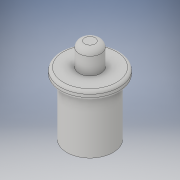
# Autodesk Inventor part: ConexionDireccionTop
Saved by Autodesk Inventor 2019 (Build 230136000, 136)
## iProperties
Created: 2019-12-22
Part Number: ConexionDireccionTop
Material: Generic
Document SubType Name: Modeling
Designer: Sergio
Density: 1 g/cm^3
Appearance: Default
Author: Sergio
Autodesk Inventor part; units mm, degrees
ref_plane "YZ Plane" through (0, 0, 0) normal (1, 0, 0) x (0, 1, 0)
ref_plane "XZ Plane" through (0, 0, 0) normal (0, 1, 0) x (-1, 0, 0)
ref_plane "XY Plane" through (0, 0, 0) normal (0, 0, 1) x (1, 0, 0)
sketch "Sketch1" plane through (0, 0, 0) normal (1, 0, 0) x (0, 1, 0)
  line L0 (30.0226, 0) -> (0.0226, 0)
  line L1 (0.0226, -8.15) -> (19.0226, -8.15)
  line L2 (19.0226, -8.15) -> (19.0226, -10.35)
  line L3 (19.0226, -10.35) -> (22.0226, -10.35)
  line L4 (22.0226, -10.35) -> (22.0226, -3.85)
  line L5 (22.0226, -3.85) -> (30.0226, -3.85)
  line L6 (30.0226, -3.85) -> (30.0226, 0)
  line L7 (0.0226, 0) -> (0.0226, -8.15)
  line L8 (50.327, 0) -> (-8.0634, 0) construction
  point P0 (0, 0)
  dimension "d0" = 3.85
  dimension "d2" = 3
  dimension "d3" = 6.5
  dimension "d4" = 8
  dimension "d5" = 30
  dimension "d7" = 8.15
  constraints: 18 end point, 4 perpendicular, 2 horizontal, 1 parallel, 1 vertical
  measures "d0" distance of L5.end L0.start
  measures "d2" distance of L2.end L3.end
  measures "d3" distance of L3.end L4.end
  measures "d4" distance of L4.end L5.end
  measures "d5" distance of L0.start L0.end
  measures "d7" distance of L0.end L1.start
revolve "Revolution1" add sketch "Sketch1" angle 360 about axis through (0, 50.327, 0) along (0, -1, 0)
fillet "Fillet1" radius 1 2 edges at (0, 22.0226, 10.35) (0, 19.0226, 10.35)
fillet "Fillet2" radius 2 1 edges at (0, 30.0226, 3.85)
body "Solid1"
